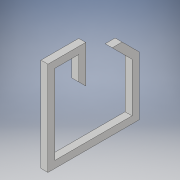
# Autodesk Inventor part: Main
Saved by Autodesk Inventor 2019 (Build 230136000, 136)
## iProperties
Created: 2018-08-02
Part Number: Main
Material: Generic
Document SubType Name: Modeling
Designer: zacha
Density: 1 g/cm^3
Appearance: Default
Author: zacha
Autodesk Inventor part; units mm, degrees
ref_plane "YZ Plane" through (0, 0, 0) normal (1, 0, 0) x (0, 1, 0)
ref_plane "XZ Plane" through (0, 0, 0) normal (0, 1, 0) x (-1, 0, 0)
ref_plane "XY Plane" through (0, 0, 0) normal (0, 0, 1) x (1, 0, 0)
sketch "Sketch1" plane through (0, 0, 0) normal (1, 0, 0) x (0, 1, 0)
  line L0 (0, 0) -> (21.5, 0)
  line L1 (21.5, 0) -> (21.5, -6.35) construction
  line L2 (21.5, -27.85) -> (0, -27.85)
  line L3 (0, -27.85) -> (0, -6.35) construction
  line L4 (21.5, 0) -> (27.85, 0)
  line L5 (27.85, 0) -> (27.85, -34.2)
  line L6 (-6.35, -34.2) -> (-6.35, -6.35) construction
  line L7 (-6.35, 0) -> (0, 0)
  line L8 (27.85, -34.2) -> (-6.35, -34.2)
  line L9 (-6.35, 0) -> (-57.15, 0)
  line L10 (-57.15, 0) -> (-57.15, -82.55)
  line L11 (-6.35, -6.35) -> (-50.8, -6.35)
  line L12 (-50.8, -6.35) -> (-50.8, -76.2)
  line L13 (-6.35, -6.35) -> (-6.35, 0) construction
  line L14 (-57.15, -82.55) -> (-3.7197, -82.55)
  line L15 (-50.8, -76.2) -> (-6.35, -76.2)
  line L16 (-6.35, -76.2) -> (11.6105, -58.2395)
  line L17 (-3.7197, -82.55) -> (11.6105, -67.2197)
  line L18 (11.6105, -58.2395) -> (11.6105, -67.2197)
  line L19 (-6.35, -34.2) -> (-6.35, -76.2) construction
  line L20 (0, -6.35) -> (21.5, -6.35)
  line L21 (0, -6.35) -> (-6.35, -6.35)
  line L22 (0, -6.35) -> (0, 0) construction
  line L23 (21.5, -6.35) -> (21.5, -27.85)
  line L24 (0, -27.85) -> (-6.35, -34.2)
  dimension "d2" = 6.35
  dimension "d4" = 6.35
  dimension "d23" = 6.35
  dimension "d24" = 50.8
  dimension "d25" = 82.55
  dimension "d26" = 6.35
  dimension "d27" = 6.35
  dimension "d28" = 6.35
  dimension "d30" = 6.35
  dimension "d31" = 25.4
  dimension "d32" = 135
  dimension "d33" = 21.5
  dimension "d34" = 6.35
  dimension "d35" = 21.5
  dimension "d36" = 24.0395
  constraints: 50 end point, 10 perpendicular, 6 horizontal, 5 parallel, 3 vertical
  measures "d2" distance of L0.end L4.end
  measures "d4" distance between parallel lines of L6 L3
  measures "d23" distance between parallel lines of L2 L8
  measures "d24" distance of L7.start L9.end
  measures "d25" distance of L9.end L10.end
  measures "d26" distance between parallel lines of L9 L11
  measures "d27" distance between parallel lines of L10 L12
  measures "d28" distance between parallel lines of L14 L15
  measures "d30" distance between parallel lines of L17 L16
  measures "d31" distance of L15.end L16.end
  measures "d32" angle of L15 L16
  measures "d33" distance between parallel lines of L2 L20
  measures "d34" distance between parallel lines of L0 L20
  measures "d35" distance between parallel lines of L3 L23
  measures "d36" distance from line of L16.end L8
extrude "Extrusion1" add sketch "Sketch1" along normal blind 6.35
equation "\"d35\" = d33"
body "Solid1"
